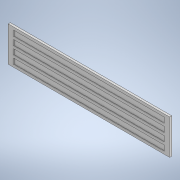
# Autodesk Inventor part: pièce1
Saved by Autodesk Inventor 2020.2 (Build 242310000, 310)
## iProperties
Created: 2020-03-03
Part Number: pièce1
Material: Générique
Document SubType Name: Modeling
Designer: anton
Density: 1 g/cm^3
Appearance: Par défaut
Author: anton
Autodesk Inventor part; units mm, degrees
ref_plane "YZ Plane" through (0, 0, 0) normal (1, 0, 0) x (0, 1, 0)
ref_plane "XZ Plane" through (0, 0, 0) normal (0, 1, 0) x (-1, 0, 0)
ref_plane "XY Plane" through (0, 0, 0) normal (0, 0, 1) x (1, 0, 0)
sketch "Esquisse1" plane through (0, 0, 0) normal (0, 0, 1) x (1, 0, 0)
  line L0 (-151.6254, 54.2183) -> (148.3746, 54.2183)
  line L1 (148.3746, 54.2183) -> (148.3746, -10.7817)
  line L2 (148.3746, -10.7817) -> (-151.6254, -10.7817)
  line L3 (-151.6254, -10.7817) -> (-151.6254, 54.2183)
  point P0 (0, 0)
  dimension "d0" = 300
  dimension "d1" = 65
  constraints: 8 end point, 2 parallel, 1 horizontal, 1 perpendicular
  measures "d0" distance of L0.start L0.end
  measures "d1" distance of L0.end L1.end
extrude "Extrusion1" add sketch "Esquisse1" along normal blind 4
sketch "Esquisse2" plane through (0, 0, 4) normal (0, 0, 1) x (1, 0, 0)
  line L0 (-141.6254, 49.2183) -> (138.3746, 49.2183)
  line L1 (138.3746, 49.2183) -> (138.3746, 39.2183)
  line L2 (138.3746, 39.2183) -> (-141.6254, 39.2183)
  line L3 (-141.6254, 39.2183) -> (-141.6254, 49.2183)
  line L4 (-141.6254, 34.2183) -> (138.3746, 34.2183)
  line L5 (138.3746, 34.2183) -> (138.3746, 24.2183)
  line L6 (138.3746, 24.2183) -> (-141.6254, 24.2183)
  line L7 (-141.6254, 24.2183) -> (-141.6254, 34.2183)
  line L8 (-141.6254, 19.2183) -> (138.3746, 19.2183)
  line L9 (138.3746, 19.2183) -> (138.3746, 9.2183)
  line L10 (138.3746, 9.2183) -> (-141.6254, 9.2183)
  line L11 (-141.6254, 9.2183) -> (-141.6254, 19.2183)
  line L12 (-141.6254, 4.2183) -> (138.3746, 4.2183)
  line L13 (138.3746, 4.2183) -> (138.3746, -5.7817)
  line L14 (138.3746, -5.7817) -> (-141.6254, -5.7817)
  line L15 (-141.6254, -5.7817) -> (-141.6254, 4.2183)
  line L16 (148.3746, 54.2183) -> (-151.6254, 54.2183) projected
  line L17 (148.3746, -10.7817) -> (148.3746, 54.2183) projected
  point P0 (0, 0)
  dimension "d4" = 5
  dimension "d5" = 10
  dimension "d6" = 5
  dimension "d7" = 10
  dimension "d8" = 5
  dimension "d9" = 10
  dimension "d10" = 5
  dimension "d11" = 10
  dimension "d12" = 280
  dimension "d13" = 10
  constraints: 32 end point, 8 parallel, 6 point on line, 4 horizontal, 4 perpendicular
  measures "d4" distance between parallel lines of L16 L0
  measures "d5" distance of L2.end L0.start
  measures "d6" distance between parallel lines of L2 L4
  measures "d7" distance of L6.end L4.start
  measures "d8" distance between parallel lines of L8 L6
  measures "d9" distance of L10.end L8.start
  measures "d10" distance between parallel lines of L10 L12
  measures "d11" distance of L14.end L12.start
  measures "d12" distance of L0.start L0.end
  measures "d13" distance between parallel lines of L17 L1
extrude "Extrusion2" cut sketch "Esquisse2" against normal blind 1
